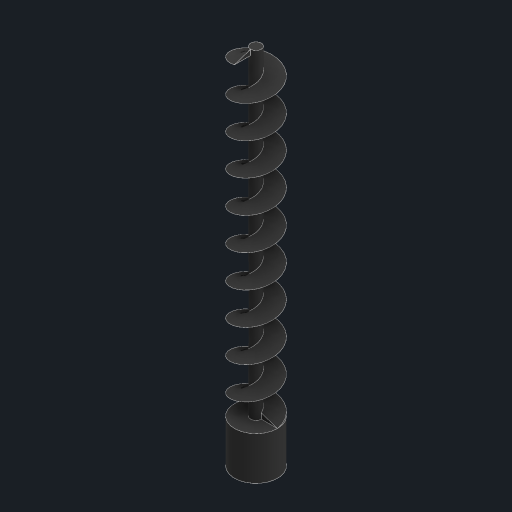
# Autodesk Inventor part: OUTK_023_Auger
Saved by Autodesk Inventor 2024.2 (Build 282272000, 272)
## iProperties
Created: 2024-12-08
Part Number: OUTK_023_Auger
Material: Rubber, Silicone
Document SubType Name: Modeling
Designer: Bryan
Density: 1.25 g/cm^3
Appearance: Rubber - Black
Author: Bryan
Autodesk Inventor part; units mm, degrees
ref_plane "YZ Plane" through (0, 0, 0) normal (1, 0, 0) x (0, 1, 0)
ref_plane "XZ Plane" through (0, 0, 0) normal (0, 1, 0) x (-1, 0, 0)
ref_plane "XY Plane" through (0, 0, 0) normal (0, 0, 1) x (1, 0, 0)
sketch "Sketch1" plane through (0, 0, 0) normal (0, 1, 0) x (-1, 0, 0)
  circle A0 centre (0, 0) radius 12.7
  line L0 (-3.6662, 6.35) -> (3.6662, 6.35)
  line L1 (3.6662, 6.35) -> (7.3323, 0)
  line L2 (7.3323, 0) -> (3.6662, -6.35)
  line L3 (3.6662, -6.35) -> (-3.6662, -6.35)
  line L4 (-3.6662, -6.35) -> (-7.3323, 0)
  line L5 (-7.3323, 0) -> (-3.6662, 6.35)
  dimension "d0" = 25.4
  dimension "d1" = 12.7
  constraints: 12 end point, 2 coincident, 1 centre point, 1 horizontal, 13 other
  measures "d0" diameter of A0
  measures "d1" distance between parallel lines of L3 L0
extrude "Extrusion1" add sketch "Sketch1" along normal blind 25.4
sketch "Sketch2" plane through (0, 25.4, 0) normal (0, 1, 0) x (1, 0, 0)
  circle A0 centre (0, 0) radius 8.4584
  constraints: 1 centre point, 1 coincident
extrude "Extrusion2" add sketch "Sketch2" against normal blind 3.175
sketch "Sketch3" plane through (0, 0, 0) normal (0, 0, 1) x (1, 0, 0)
  line L0 (12.7, 25.4) -> (-12.7, 25.4) projected
  line L1 (-3.175, 31.75) -> (3.175, 31.75)
  line L2 (3.175, 31.75) -> (3.175, 25.4)
  line L3 (3.175, 25.4) -> (-3.175, 25.4)
  line L4 (-3.175, 25.4) -> (-3.175, 31.75)
  line L5 (3.175, 28.575) -> (12.7, 25.4)
  point P0 (0, 0)
  point P1 (0, 31.75)
  point P2 (0, 25.4)
  dimension "d6" = 6.35
  constraints: 10 end point, 3 midpoint, 2 parallel, 2 perpendicular, 1 horizontal, 1 point on line, 1 vertical alignment
  measures "d6" distance of L2.end L3.end
coil "Coil1" sketch "Sketch3" operation add axis through (0, -10, 0) along (0, 1, 0) pitch 19.05 turns 9.75 hand right contours L0 L2 L5
sketch "Sketch4" plane through (0, 25.4, 0) normal (0, 1, 0) x (1, 0, 0)
  circle A0 centre (0, 0) radius 3.175
  dimension "d15" = 6.35
  constraints: 1 centre point, 1 coincident
  measures "d15" diameter of A0
extrude "Extrusion3" add sketch "Sketch4" along normal up to surface (188.9125 mm away)
body "Solid1"
